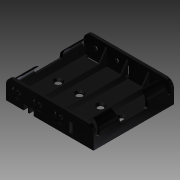
# Autodesk Inventor part: 배터리 홀더
Saved by Autodesk Inventor 2015 (Build 190159000, 159)
## iProperties
Created: 2018-01-06
Part Number: 배터리 홀더
Material: ABS 플라스틱
Document SubType Name: Modeling
Designer: choi jong in
Density: 1.06 g/cm^3
Appearance: 광택 - 검은색
Author: choi jong in
Autodesk Inventor part; units mm, degrees
ref_plane "YZ Plane" through (0, 0, 0) normal (1, 0, 0) x (0, 1, 0)
ref_plane "XZ Plane" through (0, 0, 0) normal (0, 1, 0) x (-1, 0, 0)
ref_plane "XY Plane" through (0, 0, 0) normal (0, 0, 1) x (1, 0, 0)
sketch "스케치1" plane through (0, 0, 0) normal (0, 1, 0) x (-1, 0, 0)
  line L0 (-31, 28.5) -> (31, 28.5)
  line L1 (31, 28.5) -> (31, -28.5)
  line L2 (31, -28.5) -> (-31, -28.5)
  line L3 (-31, -28.5) -> (-31, 28.5)
  line L4 (-31, 28.5) -> (31, -28.5) construction
  line L5 (31, 28.5) -> (-31, -28.5) construction
  point P0 (0, 0)
  dimension "d0" = 62
  dimension "d1" = 57
  constraints: 12 end point, 2 midpoint, 2 parallel, 1 horizontal, 1 perpendicular
  measures "d0" distance of L1.end L2.end
  measures "d1" distance of L0.end L1.end
extrude "돌출1" add sketch "스케치1" along normal blind 1.5
sketch "스케치2" plane through (-31, 0, 28.5) normal (0, 0, 1) x (1, 0, 0)
  line L0 (62, 0) -> (0, 0) projected
  line L1 (62, 0) -> (0, 0) projected
  line L2 (62, 0) -> (62, 1.5) projected
  line L3 (0, 1.5) -> (62, 1.5) projected
  line L4 (0, 0) -> (0, 1.5) projected
  line L5 (0, 0) -> (62, 0)
  line L6 (62, 0) -> (62, 15)
  line L7 (62, 15) -> (0, 15)
  line L8 (0, 15) -> (0, 0)
  point P0 (31, 0)
  dimension "d4" = 15
  constraints: 8 end point, 2 parallel, 1 collinear, 1 horizontal, 1 perpendicular
  measures "d4" distance of L7.end L1.end
extrude "돌출2" add sketch "스케치2" against normal blind 2 contours L3 L8 L7 L6
fillet "모깎기1" radius 5 2 edges at (31, 15, 27.5) (-31, 15, 27.5)
mirror "대칭1" about plane through (0, 0, 0) normal (0, 0, 1) of "모깎기1", "돌출2"
sketch "스케치3" plane through (-31, 0, 26.5) normal (0, 0, -1) x (-1, 0, 0)
  line L0 (0, 1.5) -> (-62, 1.5) projected
  line L1 (-62, 0) -> (-62, 10) projected
  line L2 (-60.5, 1.5) -> (-60.5, 8.5)
  line L3 (-57, 15) -> (-5, 15) construction
  arc A0 (-57, 15) -> (-62, 10) centre (-57, 10) ccw construction
  arc A1 (-56.0981, 15) -> (-62, 10) centre (-51.5703, 3.6722) ccw
  arc A2 (-56.0981, 15) -> (-60.5, 8.5) centre (-53.5, 8.5) ccw
  point P0 (-31, 0)
  dimension "d9" = 8.5
  dimension "d10" = 7
  dimension "d11" = 7
  constraints: 4 point on circle, 2 centre point, 2 end point, 2 point on line, 2 tangent, 1 vertical
  measures "d9" distance from line of L1 A2.centre
  measures "d10" radius of A2
  measures "d11" distance from line of L0 A2.centre
extrude "돌출3" add sketch "스케치3" along normal up to next
fillet "모깎기2" radius 2 1 edges at (31, 10, 0)
mirror "대칭2" about plane through (0, 0, 0) normal (1, 0, 0) of "모깎기2", "돌출3"
sketch "스케치4" plane through (31, 0, 28.5) normal (1, 0, 0) x (0, 0, -1)
  line L0 (2, 15) -> (2, 10) projected
  line L1 (2, 15) -> (5.4106, 15)
  line L2 (5.4106, 15) -> (4, 7)
  line L3 (4, 7) -> (2, 7)
  line L4 (2, 7) -> (2, 15)
  line L5 (57, 0) -> (0, 0) projected
  point P0 (28.5, 0)
  dimension "d15" = 2
  dimension "d16" = 7
  dimension "d20" = 100
  constraints: 8 end point, 2 vertical, 1 horizontal, 1 parallel
  measures "d15" distance of L2.end L3.end
  measures "d16" distance between parallel lines of L3 L5
  measures "d20" angle of L2 L3
extrude "돌출4" cut sketch "스케치4" against normal through all
fillet "모깎기3" radius 1 2 edges at (30.25, 7, 24.5) (-30.25, 7, 24.5)
mirror "대칭3" about plane through (0, 0, 0) normal (0, 0, 1) of "돌출4", "모깎기3"
sketch "스케치5" plane through (-31, 0, -28.5) normal (-1, 0, 0) x (0, 0, 1)
  line L0 (17.5894, 15) -> (19, 7)
  line L1 (19, 7) -> (38, 7)
  line L2 (38, 7) -> (39.4106, 15)
  line L3 (39.4106, 15) -> (17.5894, 15)
  line L4 (51.5894, 15) -> (5.4106, 15) projected
  line L5 (3.1609, 7) -> (2, 7) projected
  line L6 (28.5, 7) -> (28.5, 0) construction
  dimension "d21" = 19
  dimension "d22" = 100
  constraints: 10 end point, 2 collinear, 2 horizontal, 1 midpoint, 1 vertical, 1 other
  measures "d21" distance of L0.end L1.end
  measures "d22" angle of L1 L0
extrude "돌출5" cut sketch "스케치5" against normal through all
fillet "모깎기4" radius 1 4 edges at (-30.25, 7, -9.5) (-30.25, 7, 9.5) (30.25, 7, 9.5) (30.25, 7, -9.5)
sketch "스케치6" plane through (0, 1.5, 0) normal (0, 1, 0) x (1, 0, 0)
  line L0 (-29.5, 26.5) -> (-29.5, -26.5) projected
  line L1 (-29.5, -26.5) -> (29.5, -26.5) projected
  line L2 (29.5, -26.5) -> (29.5, 26.5) projected
  line L3 (29.5, 26.5) -> (-29.5, 26.5) projected
  line L4 (15.5, 26.5) -> (15.5, -26.5)
  line L5 (14.5, 26.5) -> (14.5, -26.5)
  line L6 (-14.5, 26.5) -> (-14.5, -26.5)
  line L7 (-15.5, 26.5) -> (-15.5, -26.5)
  line L8 (0.5, 26.5) -> (0.5, -26.5)
  line L9 (-0.5, 26.5) -> (-0.5, -26.5)
  line L10 (0, 30.5197) -> (0, -30.5197) construction
  point P0 (0, 0)
  point P1 (0, 0)
  dimension "d26" = 14
  dimension "d27" = 14
  dimension "d28" = 14
  dimension "d29" = 14
  dimension "d111" = 1
  dimension "d112" = 1
  constraints: 14 end point, 12 point on line, 4 perpendicular, 3 vertical, 1 coincident, 1 midpoint
  measures "d26" distance between parallel lines of L2 L4
  measures "d27" distance between parallel lines of L0 L7
  measures "d28" distance between parallel lines of L8 L5
  measures "d29" distance between parallel lines of L6 L9
  measures "d111" distance between parallel lines of L6 L7
  measures "d112" distance between parallel lines of L8 L9
extrude "돌출6" add sketch "스케치6" along normal up to surface (13.5 mm away) contours L3 L6 L1 L7 | L3 L8 L1 L9 | L3 L4 L1 L5
sketch "스케치7" plane through (-15.5, 1.5, -26.5) normal (-1, 0, 0) x (0, 0, 1)
  line L0 (53, 13.5) -> (0, 13.5) projected
  line L1 (0, 0) -> (0, 13.5) projected
  line L2 (53, 0) -> (0, 0) projected
  line L3 (53, 13.5) -> (53, 0) projected
  line L4 (0, 11.5) -> (5, 4)
  line L5 (5, 4) -> (48, 4)
  line L6 (48, 4) -> (53, 11.5)
  point P0 (26.5, -1.5)
  dimension "d33" = 5
  dimension "d34" = 5
  dimension "d35" = 4
  dimension "d36" = 2
  dimension "d37" = 2
  constraints: 6 end point, 2 point on line, 1 horizontal
  measures "d33" distance from line of L1 L4.end
  measures "d34" distance from line of L3 L5.end
  measures "d35" distance between parallel lines of L2 L5
  measures "d36" distance from line of L0 L4.start
  measures "d37" distance from line of L0 L6.end
extrude "돌출7" cut sketch "스케치7" against normal up to surface (31 mm away) contours L3 L6 L5 L4 L1 L0
sketch "스케치8" plane through (0, 0, 0) normal (0, -1, 0) x (1, 0, 0)
  line L0 (-28, -25) -> (28, -25)
  line L1 (28, -25) -> (28, -27)
  line L2 (28, -27) -> (-28, -27)
  line L3 (-28, -27) -> (-28, -25)
  line L4 (-31, -28.5) -> (31, -28.5) projected
  line L5 (-31, 28.5) -> (-31, -28.5) projected
  line L6 (31, -28.5) -> (31, 28.5) projected
  point P0 (0, 0)
  dimension "d40" = 2
  dimension "d41" = 1.5
  dimension "d42" = 3
  dimension "d43" = 3
  constraints: 8 end point, 2 parallel, 1 horizontal, 1 perpendicular
  measures "d40" distance of L2.end L0.start
  measures "d41" distance between parallel lines of L4 L2
  measures "d42" distance between parallel lines of L5 L3
  measures "d43" distance between parallel lines of L6 L1
extrude "돌출8" cut sketch "스케치8" against normal blind 0.5
sketch "스케치9" plane through (0, 0.5, 0) normal (0, -1, 0) x (1, 0, 0)
  line L0 (28, -25) -> (28, -27) projected
  line L1 (28, -25) -> (19, -25)
  line L2 (19, -25) -> (19, -27)
  line L3 (19, -27) -> (28, -27)
  line L4 (28, -27) -> (28, -25)
  line L5 (-28, -27) -> (-28, -25) projected
  line L6 (-28, -27) -> (-19, -27)
  line L7 (-19, -27) -> (-19, -25)
  line L8 (-19, -25) -> (-28, -25)
  line L9 (-28, -25) -> (-28, -27)
  point P0 (0, 0)
  dimension "d46" = 9
  dimension "d47" = 9
  constraints: 16 end point, 4 parallel, 2 horizontal, 2 perpendicular
  measures "d46" distance of L3.end L2.end
  measures "d47" distance of L8.end L7.end
extrude "돌출9" cut sketch "스케치9" against normal up to surface (1 mm away)
sketch "스케치10" plane through (-0.5, 1.5, -26.5) normal (-1, 0, 0) x (0, 0, 1)
  line L0 (0, 8) -> (2, 8)
  line L1 (2, 8) -> (2, 1)
  line L2 (2, 1) -> (0, 1)
  line L3 (0, 1) -> (0, 8)
  line L4 (53, 0) -> (0, 0) projected
  line L5 (0, 0) -> (0, 11.5) projected
  point P0 (26.5, -1.5)
  dimension "d50" = 7
  dimension "d51" = 1
  dimension "d52" = 2
  constraints: 8 end point, 2 parallel, 1 collinear, 1 horizontal, 1 perpendicular
  measures "d50" distance of L0.end L1.end
  measures "d51" distance between parallel lines of L4 L2
  measures "d52" distance of L0.start L0.end
extrude "돌출10" cut sketch "스케치10" against normal up to surface (1 mm away)
sketch "스케치11" plane through (-26, 15, -26.5) normal (0, 0, 1) x (1, 0, 0)
  line L0 (24.75, -5.5) -> (27.25, -5.5)
  line L1 (27.25, -5.5) -> (27.25, -12.5)
  line L2 (27.25, -12.5) -> (24.75, -12.5)
  line L3 (24.75, -12.5) -> (24.75, -5.5)
  line L4 (25.5, -5.5) -> (26.5, -5.5) projected
  line L5 (25.5, -12.5) -> (26.5, -12.5) projected
  line L6 (26, -1.762) -> (26, -12.5) construction
  point P0 (26, -15)
  dimension "d55" = 2.5
  constraints: 10 end point, 2 collinear, 2 parallel, 1 horizontal, 1 midpoint, 1 perpendicular, 1 other
  measures "d55" distance between parallel lines of L1 L3
extrude "돌출11" cut sketch "스케치11" against normal up to surface (2 mm away)
sketch "스케치12" plane through (14.5, 1.5, -26.5) normal (-1, 0, 0) x (0, 0, 1)
  line L0 (51, 8) -> (53, 8)
  line L1 (53, 8) -> (53, 1)
  line L2 (53, 1) -> (51, 1)
  line L3 (51, 1) -> (51, 8)
  line L4 (53, 11.5) -> (53, 0) projected
  line L5 (53, 0) -> (0, 0) projected
  point P0 (26.5, -1.5)
  dimension "d58" = 2
  dimension "d59" = 7
  dimension "d60" = 1
  constraints: 8 end point, 2 parallel, 1 collinear, 1 horizontal, 1 perpendicular
  measures "d58" distance of L1.end L2.end
  measures "d59" distance of L0.end L1.end
  measures "d60" distance between parallel lines of L5 L2
extrude "돌출12" cut sketch "스케치12" against normal up to surface (1 mm away)
sketch "스케치13" plane through (-31, 0, 26.5) normal (0, 0, -1) x (-1, 0, 0)
  line L0 (-47.25, 9.5) -> (-44.75, 9.5)
  line L1 (-44.75, 9.5) -> (-44.75, 2.5)
  line L2 (-44.75, 2.5) -> (-47.25, 2.5)
  line L3 (-47.25, 2.5) -> (-47.25, 9.5)
  line L4 (-45.5, 2.5) -> (-46.5, 2.5) projected
  line L5 (-45.5, 9.5) -> (-46.5, 9.5) projected
  line L6 (-46, 12.9661) -> (-46, 2.5) construction
  point P0 (-31, 0)
  dimension "d63" = 2.5
  constraints: 10 end point, 2 collinear, 2 parallel, 1 horizontal, 1 midpoint, 1 perpendicular, 1 other
  measures "d63" distance of L1.end L2.end
extrude "돌출13" cut sketch "스케치13" against normal up to surface (2 mm away)
sketch "스케치14" plane through (0, 1.5, 0) normal (0, 1, 0) x (1, 0, 0)
  line L0 (-4.5, -26.5) -> (-10.5, -26.5)
  line L1 (-10.5, -26.5) -> (-10.5, -24.5)
  line L2 (-10.5, -24.5) -> (-4.5, -24.5)
  line L3 (-4.5, -24.5) -> (-4.5, -26.5)
  line L4 (-19.5, -26.5) -> (-25.5, -26.5)
  line L5 (-25.5, -26.5) -> (-25.5, -24.5)
  line L6 (-25.5, -24.5) -> (-19.5, -24.5)
  line L7 (-19.5, -24.5) -> (-19.5, -26.5)
  line L8 (-14.5, -21.5) -> (-14.5, -26.5) projected
  line L9 (-15.5, -26.5) -> (-15.5, -21.5) projected
  line L10 (-26, -26.5) -> (26, -26.5) projected
  point P0 (0, 0)
  dimension "d66" = 6
  dimension "d67" = 6
  dimension "d68" = 2
  dimension "d69" = 4
  dimension "d70" = 4
  constraints: 16 end point, 4 parallel, 2 horizontal, 2 perpendicular, 2 point on line, 1 collinear
  measures "d66" distance of L1.end L2.end
  measures "d67" distance of L5.end L6.end
  measures "d68" distance of L2.end L0.start
  measures "d69" distance between parallel lines of L8 L1
  measures "d70" distance between parallel lines of L9 L7
extrude "돌출14" cut sketch "스케치14" against normal up to surface (1.5 mm away)
sketch "스케치15" plane through (0, 0, 0) normal (0, -1, 0) x (1, 0, 0)
  line L0 (-11.5, 24.5) -> (-14.5, 24.5)
  line L1 (-14.5, 24.5) -> (-14.5, 26.5)
  line L2 (-14.5, 26.5) -> (-11.5, 26.5)
  line L3 (-11.5, 26.5) -> (-11.5, 24.5)
  line L4 (-18.5, 24.5) -> (-15.5, 24.5)
  line L5 (-15.5, 24.5) -> (-15.5, 26.5)
  line L6 (-15.5, 26.5) -> (-18.5, 26.5)
  line L7 (-18.5, 26.5) -> (-18.5, 24.5)
  line L8 (-4.5, 24.5) -> (-10.5, 24.5) projected
  line L9 (-19.5, 24.5) -> (-25.5, 24.5) projected
  line L10 (-10.5, 26.5) -> (-4.5, 26.5) projected
  line L11 (-25.5, 26.5) -> (-19.5, 26.5) projected
  line L12 (-10.5, 24.5) -> (-10.5, 26.5) projected
  line L13 (-19.5, 26.5) -> (-19.5, 24.5) projected
  line L14 (-14.5, -26.5) -> (-14.5, 26.5) projected
  line L15 (-15.5, 26.5) -> (-15.5, -26.5) projected
  point P0 (0, 0)
  dimension "d73" = 1
  dimension "d74" = 1
  constraints: 16 end point, 6 collinear, 4 parallel, 2 horizontal, 2 perpendicular
  measures "d73" distance between parallel lines of L12 L3
  measures "d74" distance between parallel lines of L13 L7
extrude "돌출15" cut sketch "스케치15" against normal up to surface (1.5 mm away)
sketch "스케치16" plane through (-31, 0, 26.5) normal (0, 0, -1) x (-1, 0, 0)
  line L0 (-19.5, 0) -> (-16.5, 0)
  line L1 (-16.5, 0) -> (-16.5, 4)
  line L2 (-16.5, 4) -> (-19.5, 4)
  line L3 (-19.5, 4) -> (-19.5, 0)
  line L4 (-15.5, 0) -> (-12.5, 0)
  line L5 (-12.5, 0) -> (-12.5, 4)
  line L6 (-12.5, 4) -> (-15.5, 4)
  line L7 (-15.5, 4) -> (-15.5, 0)
  line L8 (-16.5, 0) -> (-19.5, 0) projected
  line L9 (-19.5, 0) -> (-19.5, 1.5) projected
  line L10 (-16.5, 0) -> (-16.5, 13) projected
  line L11 (-12.5, 0) -> (-12.5, 1.5) projected
  line L12 (-12.5, 0) -> (-15.5, 0) projected
  line L13 (-15.5, 13) -> (-15.5, 0) projected
  point P0 (-31, 0)
  dimension "d77" = 4
  dimension "d78" = 4
  constraints: 16 end point, 6 collinear, 4 parallel, 2 horizontal, 2 perpendicular
  measures "d77" distance of L2.end L0.start
  measures "d78" distance of L4.end L5.end
extrude "돌출16" cut sketch "스케치16" against normal up to surface (2 mm away)
sketch "스케치17" plane through (-26, 15, 28.5) normal (0, 0, 1) x (1, 0, 0)
  line L0 (27.25, -12.5) -> (26.5, -12.5) projected
  line L1 (26.5, -12.5) -> (26.5, -13.5) projected
  line L2 (40.5, -13.5) -> (26.5, -13.5) projected
  line L3 (40.5, -13.5) -> (40.5, -2) projected
  line L4 (40.5, -2) -> (41.5, -2) projected
  line L5 (41.5, -2) -> (41.5, -13.5) projected
  line L6 (45, -13.5) -> (41.5, -13.5) projected
  line L7 (54, -13.5) -> (45, -13.5) projected
  line L8 (55.5, -13.5) -> (54, -13.5) projected
  line L9 (55.5, -13.5) -> (55.5, -8) projected
  line L10 (57, -8) -> (55.5, -8) projected
  line L11 (57, -8) -> (57, -5) projected
  arc A0 (57, -5) -> (52, 0) centre (52, -5) ccw projected
  line L12 (0, 0) -> (52, 0) projected
  arc A1 (0, 0) -> (-5, -5) centre (0, -5) ccw projected
  line L13 (-5, -5) -> (-5, -8) projected
  line L14 (-3.5, -8) -> (-5, -8) projected
  line L15 (-3.5, -8) -> (-3.5, -13.5) projected
  line L16 (-2, -13.5) -> (-3.5, -13.5) projected
  line L17 (7, -13.5) -> (-2, -13.5) projected
  line L18 (10.5, -13.5) -> (7, -13.5) projected
  line L19 (10.5, -13.5) -> (10.5, -2) projected
  line L20 (10.5, -2) -> (11.5, -2) projected
  line L21 (11.5, -2) -> (11.5, -13.5) projected
  line L22 (25.5, -13.5) -> (11.5, -13.5) projected
  line L23 (25.5, -13.5) -> (25.5, -12.5) projected
  line L24 (25.5, -12.5) -> (24.75, -12.5) projected
  line L25 (24.75, -12.5) -> (24.75, -5.5) projected
  line L26 (24.75, -5.5) -> (25.5, -5.5) projected
  line L27 (25.5, -5.5) -> (25.5, -2) projected
  line L28 (25.5, -2) -> (26.5, -2) projected
  line L29 (26.5, -2) -> (26.5, -5.5) projected
  line L30 (26.5, -5.5) -> (27.25, -5.5) projected
  line L31 (27.25, -5.5) -> (27.25, -12.5) projected
  circle A2 centre (3.5, -6.5) radius 7 construction
  circle A3 centre (18.5, -6.5) radius 7 construction
  circle A4 centre (33.5, -6.5) radius 7 construction
  circle A5 centre (3.5, -6.5) radius 4
  circle A6 centre (18.5, -6.5) radius 4
  circle A7 centre (33.5, -6.5) radius 4
  point P0 (26, -15)
  dimension "d81" = 14
  dimension "d82" = 14
  dimension "d83" = 14
  dimension "d84" = 8
  dimension "d85" = 8
  dimension "d86" = 8
  constraints: 6 centre point, 6 tangent, 3 coincident
  measures "d81" diameter of A2
  measures "d82" diameter of A3
  measures "d83" diameter of A4
  measures "d84" diameter of A5
  measures "d85" diameter of A6
  measures "d86" diameter of A7
extrude "돌출17" cut sketch "스케치17" against normal blind 0.5 contours A5 | A6 | A7
sketch "스케치18" plane through (31, 0, -28.5) normal (0, 0, -1) x (-1, 0, 0)
  line L0 (42.5, 4) -> (45.5, 4) projected
  line L1 (45.5, 4) -> (45.5, 13) projected
  line L2 (46.5, 13) -> (45.5, 13) projected
  line L3 (46.5, 13) -> (46.5, 4) projected
  line L4 (46.5, 4) -> (49.5, 4) projected
  line L5 (49.5, 4) -> (49.5, 1.5) projected
  line L6 (50.5, 1.5) -> (49.5, 1.5) projected
  line L7 (50.5, 1.5) -> (50.5, 0) projected
  line L8 (56.5, 0) -> (50.5, 0) projected
  line L9 (56.5, 1.5) -> (56.5, 0) projected
  line L10 (60.5, 1.5) -> (56.5, 1.5) projected
  line L11 (60.5, 1.5) -> (60.5, 7) projected
  line L12 (60.5, 7) -> (62, 7) projected
  line L13 (62, 7) -> (62, 10) projected
  arc A0 (62, 10) -> (57, 15) centre (57, 10) ccw projected
  line L14 (57, 15) -> (5, 15) projected
  arc A1 (5, 15) -> (0, 10) centre (5, 10) ccw projected
  line L15 (0, 10) -> (0, 7) projected
  line L16 (0, 7) -> (1.5, 7) projected
  line L17 (1.5, 7) -> (1.5, 1.5) projected
  line L18 (15.5, 1.5) -> (1.5, 1.5) projected
  line L19 (15.5, 1.5) -> (15.5, 2.5) projected
  line L20 (15.5, 2.5) -> (14.75, 2.5) projected
  line L21 (14.75, 2.5) -> (14.75, 9.5) projected
  line L22 (14.75, 9.5) -> (15.5, 9.5) projected
  line L23 (15.5, 9.5) -> (15.5, 13) projected
  line L24 (16.5, 13) -> (15.5, 13) projected
  line L25 (16.5, 13) -> (16.5, 9.5) projected
  line L26 (16.5, 9.5) -> (17.25, 9.5) projected
  line L27 (17.25, 9.5) -> (17.25, 2.5) projected
  line L28 (17.25, 2.5) -> (16.5, 2.5) projected
  line L29 (16.5, 2.5) -> (16.5, 1.5) projected
  line L30 (30.5, 1.5) -> (16.5, 1.5) projected
  line L31 (30.5, 1.5) -> (30.5, 13) projected
  line L32 (31.5, 13) -> (30.5, 13) projected
  line L33 (31.5, 13) -> (31.5, 1.5) projected
  line L34 (35.5, 1.5) -> (31.5, 1.5) projected
  line L35 (35.5, 1.5) -> (35.5, 0) projected
  line L36 (41.5, 0) -> (35.5, 0) projected
  line L37 (41.5, 1.5) -> (41.5, 0) projected
  line L38 (42.5, 1.5) -> (41.5, 1.5) projected
  line L39 (42.5, 1.5) -> (42.5, 4) projected
  line L40 (29.75, 2.5) -> (29.75, 9.5) projected
  line L41 (29.75, 9.5) -> (32.25, 9.5) projected
  line L42 (32.25, 9.5) -> (32.25, 2.5) projected
  line L43 (32.25, 2.5) -> (29.75, 2.5) projected
  line L44 (0, 0) -> (0, 10) projected
  line L45 (62, 0) -> (0, 0) projected
  line L46 (62, 0) -> (62, 10) projected
  arc A2 (62, 10) -> (57, 15) centre (57, 10) ccw projected
  line L47 (5, 15) -> (57, 15) projected
  arc A3 (5, 15) -> (0, 10) centre (5, 10) ccw projected
  circle A4 centre (53.5, 8.5) radius 7 construction
  line L48 (46.5, 1.5) -> (50, 1.5) projected
  circle A5 centre (38.5, 8.5) radius 7 construction
  circle A6 centre (8.5, 8.5) radius 7 construction
  circle A7 centre (8.5, 8.5) radius 4
  circle A8 centre (38.5, 8.5) radius 4
  circle A9 centre (53.5, 8.5) radius 4
  point P0 (31, 0)
  dimension "d89" = 14
  dimension "d90" = 14
  dimension "d91" = 14
  dimension "d92" = 8
  dimension "d93" = 8
  dimension "d94" = 8
  constraints: 6 centre point, 6 tangent, 3 coincident
  measures "d89" diameter of A4
  measures "d90" diameter of A5
  measures "d91" diameter of A6
  measures "d92" diameter of A7
  measures "d93" diameter of A8
  measures "d94" diameter of A9
extrude "돌출18" cut sketch "스케치18" against normal blind 0.5 contours A7 | A8 | A9
sketch "스케치19" plane through (-26, 15, 28.5) normal (0, 0, 1) x (1, 0, 0)
  circle A0 centre (3.5, -6.5) radius 4 projected
  circle A1 centre (18.5, -6.5) radius 4 projected
  circle A2 centre (33.5, -6.5) radius 4 projected
  point P0 (26, -15)
hole "구멍1" at (-7.5, 8.5, 28.5) at (-22.5, 8.5, 28.5) at (7.5, 8.5, 28.5) direction (0, 0, -1) diameter 3 end up to surface
sketch "스케치20" plane through (22.5, 8.5, -28) normal (0, 0, -1) x (-1, 0, 0)
  circle A0 centre (0, 0) radius 4 projected
  circle A1 centre (30, 0) radius 4 projected
  circle A2 centre (45, 0) radius 4 projected
  point P0 (22.5, -8.5)
hole "구멍2" at (22.5, 8.5, -28) at (-7.5, 8.5, -28) at (-22.5, 8.5, -28) direction (0, 0, 1) diameter 3 end up to surface
sketch "스케치21" plane through (0, 1.5, 0) normal (0, 1, 0) x (1, 0, 0)
  line L0 (-29.5, 26.5) -> (-29.5, -26.5) projected
  line L1 (-29.5, 0) -> (-15.5, 0) construction
  point P0 (0, 0)
  point P1 (-22.5, 0)
  point P2 (-22.5, 0)
  dimension "d114" = 14
  constraints: 2 end point, 2 midpoint, 1 coincident, 1 horizontal
  measures "d114" distance of L1.start L1.end
hole "구멍3" at (-22.5, 1.5, 0) direction (0, -1, 0) diameter 4 end through all
pattern_linear "직사각형 패턴1" count 4 spacing 15 along (1, 0, 0) of "구멍3"
chamfer "모따기1" distance 1 angle 45 4 edges at (-22.5, 1.5, -2) (-7.5, 1.5, -2) (7.5, 1.5, -2) (22.5, 1.5, -2)
